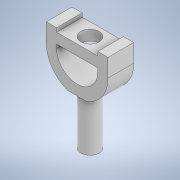
# Autodesk Inventor part: Universal joint
Saved by Autodesk Inventor 2021 (Build 250183000, 183)
## iProperties
Created: 2024-12-12
Part Number: Universal joint
Material: Generic
Document SubType Name: Modeling
Designer: 24lucsil
Density: 1 g/cm^3
Appearance: Default
Author: 24lucsil
Autodesk Inventor part; units mm, degrees
ref_plane "YZ Plane" through (0, 0, 0) normal (1, 0, 0) x (0, 1, 0)
ref_plane "XZ Plane" through (0, 0, 0) normal (0, 1, 0) x (-1, 0, 0)
ref_plane "XY Plane" through (0, 0, 0) normal (0, 0, 1) x (1, 0, 0)
sketch "Sketch1" plane through (0, 0, 0) normal (0, 1, 0) x (-1, 0, 0)
  circle A0 centre (0, 0) radius 3.55
  circle A1 centre (0, 0) radius 2.8
  line L0 (0, -2.8) -> (0, -1.9)
  line L1 (0, 2.8) -> (0, 1.9)
  line L2 (2.0567, 1.9) -> (-2.0567, 1.9)
  line L3 (-2.0567, -1.9) -> (2.0567, -1.9)
  dimension "d0" = 7.1
  dimension "d1" = 5.6
  dimension "d2" = 0.9
  dimension "d3" = 0.9
  dimension "d4" = 4.1134
  dimension "d5" = 4.1134
  constraints: 8 end point, 6 point on circle, 2 centre point, 2 coincident, 2 vertical, 1 horizontal, 1 parallel
  measures "d0" diameter of A0
  measures "d1" diameter of A1
  measures "d2" distance of L0.start L0.end
  measures "d3" distance of L1.start L1.end
  measures "d4" distance of L3.start L3.end
  measures "d5" distance of L2.start L2.end
extrude "Extrusion1" add sketch "Sketch1" along normal blind 8.5 contours A0 | L2 L1 A1 | A1 L0 L3 | L1 L2 A1 | A1 L3 L0
sketch "Sketch2" plane through (0, 8.5, 0) normal (0, 1, 0) x (1, 0, 0)
  arc A0 (-2.0567, 1.9) -> (-2.0567, -1.9) centre (0, 0) ccw projected
  circle A1 centre (0, 0) radius 3.55
  dimension "d8" = 7.1
  constraints: 1 centre point, 1 coincident
  measures "d8" diameter of A1
extrude "Extrusion2" add sketch "Sketch2" along normal blind 11.5
sketch "Sketch3" plane through (0, 0, 0) normal (0, 0, 1) x (1, 0, 0)
  line L0 (3.55, 20) -> (-3.55, 20) construction
  line L1 (0, 20) -> (0, 32) construction
  line L2 (0, 32) -> (-12, 32) construction
  line L3 (0, 32) -> (12, 32) construction
  arc A0 (-12, 32) -> (-3.55, 20) centre (0.4988, 31.8261) ccw
  arc A1 (3.55, 20) -> (12, 32) centre (-0.4988, 31.8261) ccw
  line L4 (-12, 32) -> (-8, 32)
  line L5 (12, 32) -> (8, 32)
  circle A2 centre (0, 32) radius 8
  line L6 (-12, 32) -> (-8, 32)
  line L7 (-8, 32) -> (-8, 39)
  line L8 (-8, 39) -> (-12, 39)
  line L9 (-12, 39) -> (-12, 32)
  line L10 (12, 32) -> (8, 32)
  line L11 (8, 32) -> (8, 39)
  line L12 (8, 39) -> (12, 39)
  line L13 (12, 39) -> (12, 32)
  line L14 (-8, 32) -> (-8, 34.0142) construction
  line L15 (-8, 39) -> (-8, 37.5) construction
  line L16 (8, 32) -> (8, 35.1588) construction
  line L17 (-8, 37.5) -> (8, 37.5)
  line L18 (8, 37.5) -> (8, 33.5)
  line L19 (8, 33.5) -> (-8, 33.5)
  line L20 (-8, 33.5) -> (-8, 37.5)
  line L21 (-3.55, 20) -> (3.55, 20)
  point P0 (0, 0)
  point P1 (8, 37.5)
  dimension "d11" = 12
  dimension "d12" = 12
  dimension "d13" = 12
  dimension "d14" = 12.5
  dimension "d15" = 12.5
  dimension "d16" = 4
  dimension "d17" = 4
  dimension "d18" = 7
  dimension "d19" = 7
  dimension "d20" = 4
  dimension "d21" = 4
  dimension "d22" = 1.5
  dimension "d23" = 1.5
  dimension "d24" = 1.5
  constraints: 42 end point, 7 equal length, 7 point on line, 5 horizontal, 4 point on circle, 3 perpendicular, 2 centre point, 1 coincident, 1 midpoint, 1 vertical, 3 other
  measures "d11" distance of L1.start L1.end
  measures "d12" distance of L1.end L2.end
  measures "d13" distance of L1.end L3.end
  measures "d14" radius of A0
  measures "d15" radius of A1
  measures "d16" distance of L2.end L4.end
  measures "d17" distance of L3.end L5.end
  measures "d18" distance of L6.end L7.end
  measures "d19" distance of L10.end L11.end
  measures "d20" distance of L11.end L12.end
  measures "d21" distance of L7.end L8.end
  measures "d22" distance of L4.end point (-8, 33.5)
  measures "d23" distance of L15.end L7.end
  measures "d24" distance of L5.end L18.end
extrude "Extrusion3" add sketch "Sketch3" along normal mid plane 10 contours L4 A2 L5 A1 L21 A0 | L9 L8 L7 L4 | L11 L12 L13 L5 | L19 L7 L17 A2 | A2 L17 L19 | A2 L17 L11 L19
sketch "Sketch4" plane through (-8, 37.5, 5) normal (0, 1, 0) x (1, 0, 0)
  circle A0 centre (8, 5) radius 3.55 projected
  circle A1 centre (8, 5) radius 3.55
  point P0 (8, 3.5)
  constraints: 1 centre point, 1 coincident
extrude "Extrusion4" cut sketch "Sketch4" against normal blind 10
body "Solid1"
